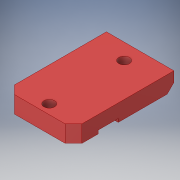
# Autodesk Inventor part: КВ33.044.202 - Прижим ремня
Saved by Autodesk Inventor 2019 (Build 230136000, 136)
## iProperties
Created: 2019-08-04
Part Number: КВ33.044.202 - Прижим ремня
Material: Пластик АБС
Document SubType Name: Modeling
Designer: Петров Иван
Density: 1.06 g/cm^3
Appearance: Гладкий — красный
Author: Петров Иван
Autodesk Inventor part; units mm, degrees
ref_plane "YZ Plane" through (0, 0, 0) normal (1, 0, 0) x (0, 1, 0)
ref_plane "XZ Plane" through (0, 0, 0) normal (0, 1, 0) x (-1, 0, 0)
ref_plane "XY Plane" through (0, 0, 0) normal (0, 0, 1) x (1, 0, 0)
sketch "Эскиз1" plane through (0, 0, 0) normal (0, 1, 0) x (-1, 0, 0)
  line L0 (17.5, -26.75) -> (-2.5, -26.75)
  line L1 (17.5, -26.75) -> (17.5, -2.5)
  line L2 (15, 0) -> (17.5, -2.5)
  line L3 (0, 0) -> (15, 0)
  line L4 (-2.5, -2.5) -> (0, 0)
  line L5 (-2.5, -26.75) -> (-2.5, -2.5)
  circle A0 centre (7.5, -2.8) radius 1.6
  circle A1 centre (7.5, -25) radius 1.6
  point P0 (7.5, -40)
  constraints: 12 end point, 2 centre point
extrude "Выдавливание1" add sketch "Эскиз1" along normal blind 5
sketch "Эскиз2" plane through (0, 0, 0) normal (0, -1, 0) x (1, 0, 0)
  line L0 (2.5, -2.5) -> (2.5, -26.75) projected
  line L1 (-17.5, -26.75) -> (-17.5, -2.5) projected
  line L2 (2.5, -7.2576) -> (-17.5, -7.2576)
  line L3 (-17.5, -7.2576) -> (-17.5, -13.2576)
  line L4 (-17.5, -13.2576) -> (2.5, -13.2576)
  line L5 (2.5, -13.2576) -> (2.5, -7.2576)
  point P0 (0, 0)
  dimension "d2" = 6
  constraints: 8 end point, 2 parallel, 2 point on line, 1 horizontal, 1 perpendicular
  measures "d2" distance of L3.end L2.end
extrude "Выдавливание2" cut sketch "Эскиз2" against normal blind 1
move faces "Перенос1" translate (0, 0, -3) faces at (-4.1667, 1.6667, -26.75)
chamfer "Фаска1" distance 2 angle 45 1 edges at (-7.5, 0, -29.75)
